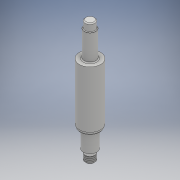
# Autodesk Inventor part: 도면2-3번
Saved by Autodesk Inventor 2018.3 (Build 223284000, 284)
## iProperties
Created: 2019-10-11
Part Number: 도면2-3번
Material: 일반
Document SubType Name: Modeling
Designer: MyTool
Density: 1 g/cm^3
Appearance: 기본값
Author: MyTool
Autodesk Inventor part; units mm, degrees
ref_plane "YZ Plane" through (0, 0, 0) normal (1, 0, 0) x (0, 1, 0)
ref_plane "XZ Plane" through (0, 0, 0) normal (0, 1, 0) x (-1, 0, 0)
ref_plane "XY Plane" through (0, 0, 0) normal (0, 0, 1) x (1, 0, 0)
sketch "스케치1" plane through (0, 0, 0) normal (1, 0, 0) x (0, 1, 0)
  line L0 (0, 0) -> (5, 0)
  line L1 (5, 0) -> (5, 11)
  line L2 (5, 11) -> (0, 11)
  line L3 (0, 11) -> (0, 0)
  line L4 (0, 11) -> (7, 11)
  line L5 (7, 11) -> (7, 30)
  line L6 (7, 30) -> (0, 30)
  line L7 (0, 30) -> (0, 11)
  line L8 (0, 30) -> (11, 30)
  line L9 (11, 30) -> (11, 92)
  line L10 (11, 92) -> (0, 92)
  line L11 (0, 92) -> (0, 30)
  line L12 (0, 92) -> (6, 92)
  line L13 (6, 92) -> (6, 119)
  line L14 (6, 119) -> (0, 119)
  line L15 (0, 119) -> (0, 92)
  line L16 (0, 119) -> (5, 119)
  line L17 (5, 119) -> (5, 127)
  line L18 (5, 127) -> (0, 127)
  line L19 (0, 127) -> (0, 119)
  dimension "d0" = 19
  dimension "d1" = 11
  dimension "d2" = 62
  dimension "d3" = 27
  dimension "d4" = 8
  dimension "d8" = 10
  dimension "d9" = 14
  dimension "d10" = 22
  dimension "d11" = 12
  dimension "d12" = 10
  constraints: 40 end point, 10 parallel, 5 horizontal, 5 perpendicular
  measures "d0" distance of L5.end L4.end
  measures "d1" distance of L0.end L1.end
  measures "d2" distance of L8.end L9.end
  measures "d3" distance of L12.end L13.end
  measures "d4" distance of L16.end L17.end
  measures "d8" diameter of L1 L3
  measures "d9" diameter of L5 L7
  measures "d10" diameter of L9 L11
  measures "d11" diameter of L13 L15
  measures "d12" diameter of L17 L19
revolve "회전1" add sketch "스케치1" angle 360 about axis through (0, 0, 92) along (0, 0, -1)
thread "스레드1" size "M10x1.5" class "6g" standard "ANSI Metric M Profile" full length
sketch "스케치2" plane through (0, 0, 0) normal (1, 0, 0) x (0, 1, 0)
  line L0 (5, 11) -> (5, 0) projected
  line L1 (5, 11) -> (5, 7.25)
  line L2 (4, 9) -> (4, 11)
  line L3 (4, 11) -> (5, 11)
  line L4 (5, 7.25) -> (4, 9)
  line L5 (0, -25.4) -> (0, 152.4) projected
  point P0 (0, 0)
  dimension "d17" = 2
  dimension "d18" = 3.75
  dimension "d19" = 1
  constraints: 8 end point, 1 perpendicular, 1 point on line, 1 vertical
  measures "d17" distance of L2.start L2.end
  measures "d18" distance of L1.end L0.start
  measures "d19" distance of L2.end L0.start
revolve "회전2" cut sketch "스케치2" angle 360 about axis through (0, 0, -10) along (0, 0, 1)
fillet "모깎기1" radius 0.6 2 edges at (0, -4, 11) (0, -4, 9)
sketch "스케치3" plane through (0, 0, 0) normal (1, 0, 0) x (0, 1, 0)
  line L0 (11, 30) -> (11, 32.0785)
  line L1 (11, 92) -> (11, 30) projected
  line L2 (9.8, 30) -> (11, 30)
  line L3 (9.8, 30) -> (11, 32.0785)
  line L4 (0, -25.4) -> (0, 152.4) projected
  point P0 (0, 0)
  dimension "d22" = 30
  dimension "d23" = 1.2
  constraints: 6 end point, 1 perpendicular, 1 point on line
  measures "d22" angle of L0 L3
  measures "d23" distance of L2.start L0.start
revolve "회전3" cut sketch "스케치3" angle 360 about axis through (0, 0, -10) along (0, 0, 1)
fillet "모깎기2" radius 4 1 edges at (0, -11, 32.0785)
fillet "모깎기3" radius 1 1 edges at (0, -9.8, 30)
fillet "모깎기4" radius 1 1 edges at (0, -6, 92)
fillet "모깎기5" radius 0.5 1 edges at (0, -5, 119)
chamfer "모따기1" distance 1 angle 45 2 edges at (0, -5, 127) (0, -5, 0)
